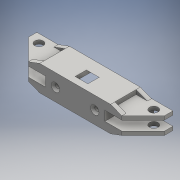
# Autodesk Inventor part: Support_GP2.C
Saved by Autodesk Inventor 2016 (Build 200138000, 138)
## iProperties
Created: 2016-09-29
Part Number: Support_GP2.C
Material: Générique
Document SubType Name: Modeling
Designer: LogOut
Density: 1 g/cm^3
Appearance: Par défaut
Author: LogOut
Autodesk Inventor part; units mm, degrees
ref_plane "YZ Plane" through (0, 0, 0) normal (1, 0, 0) x (0, 1, 0)
ref_plane "XZ Plane" through (0, 0, 0) normal (0, 1, 0) x (-1, 0, 0)
ref_plane "XY Plane" through (0, 0, 0) normal (0, 0, 1) x (1, 0, 0)
sketch "Esquisse1" plane through (0, 0, 0) normal (0, 0, 1) x (1, 0, 0)
  line L0 (-64, 14) -> (64, 14)
  line L1 (64, 14) -> (64, -14)
  line L2 (64, -14) -> (-64, -14)
  line L3 (-64, -14) -> (-64, 14)
  point P0 (0, 0)
  dimension "d0" = 128
  dimension "d1" = 28
  dimension "d2" = 14
  dimension "d3" = 64
  constraints: 8 end point, 2 parallel, 1 horizontal, 1 perpendicular
  measures "d0" distance of L0.start L0.end
  measures "d1" distance of L2.end L0.start
  measures "d2" distance from line of point (0, 0) L0
  measures "d3" distance from line of point (0, 0) L1
extrude "Extrusion1" add sketch "Esquisse1" along normal blind 28
sketch "Esquisse2" plane through (-64, 14, 0) normal (0, 1, 0) x (1, 0, 0)
  line L0 (40, -22) -> (88, -22)
  line L1 (88, -22) -> (88, -6)
  line L2 (88, -6) -> (40, -6)
  line L3 (40, -6) -> (40, -22)
  line L4 (0, 0) -> (128, 0) projected
  line L5 (0, 0) -> (0, -28) projected
  line L6 (128, -28) -> (0, -28) projected
  line L7 (128, 0) -> (128, -28) projected
  point P0 (64, 0)
  dimension "d6" = 40
  dimension "d7" = 48
  dimension "d8" = 40
  dimension "d9" = 6
  dimension "d10" = 6
  dimension "d11" = 16
  constraints: 8 end point, 2 parallel, 1 horizontal, 1 perpendicular
  measures "d6" distance between parallel lines of L5 L3
  measures "d7" distance between parallel lines of L1 L3
  measures "d8" distance between parallel lines of L7 L1
  measures "d9" distance between parallel lines of L4 L2
  measures "d10" distance between parallel lines of L6 L0
  measures "d11" distance of L2.end L0.start
extrude "Extrusion2" cut sketch "Esquisse2" against normal blind 24 contours L3 L2 L1 L0
ref_plane "Plan de construction1" through (-24, 14, 14) normal (0, 0, 1) x (1, 0, 0)
sketch "Esquisse3" plane through (-24, 14, 14) normal (0, 0, 1) x (1, 0, 0)
  line L0 (112.7171, 2) -> (72, 2)
  line L1 (72, 2) -> (52, -18)
  line L2 (-4, -18) -> (-24, 2)
  line L3 (-24, 2) -> (-79.3521, 2)
  line L4 (88, -28) -> (-40, -28) projected
  line L5 (112.7171, 2) -> (112.7171, -53.3012)
  line L6 (112.7171, -53.3012) -> (-79.3521, -53.3012)
  line L7 (-79.3521, -53.3012) -> (-79.3521, 2)
  line L8 (-4, -18) -> (-4, -28)
  line L9 (-40, -28) -> (88, -28) projected
  line L10 (-4, -28) -> (52, -28)
  line L11 (52, -28) -> (52, -18)
  point P0 (24, -14)
  point P1 (54.2399, -28)
  point P2 (-6.2399, -28)
  dimension "d22" = 30
  dimension "d23" = 20
  dimension "d24" = 20
  dimension "d25" = 56
  dimension "d26" = 28
  dimension "d27" = 28
  dimension "d28" = 20
  dimension "d29" = 20
  constraints: 20 end point, 5 perpendicular, 4 point on line, 1 collinear, 1 horizontal, 1 vertical
  measures "d22" distance between parallel lines of L3 L4
  measures "d23" horizontal distance of L2.start L2.end
  measures "d24" horizontal distance of L2.start L2.end
  measures "d25" distance between parallel lines of L11 L8
  measures "d26" distance from line of point (24, -14) L11
  measures "d27" distance from line of point (24, -14) L8
  measures "d28" horizontal distance of L0.end L1.end
  measures "d29" horizontal distance of L0.end L1.end
extrude "Extrusion3" cut sketch "Esquisse3" along normal mid plane 8
sketch "Esquisse4" plane through (0, 0, 28) normal (0, 0, 1) x (1, 0, 0)
  line L0 (88.7171, 16) -> (48, 16)
  line L1 (48, 16) -> (28, -4)
  line L2 (-28, -4) -> (-48, 16)
  line L3 (-48, 16) -> (-103.3521, 16)
  line L4 (88.7171, 16) -> (88.7171, -39.3012)
  line L5 (88.7171, -39.3012) -> (-103.3521, -39.3012)
  line L6 (-103.3521, -39.3012) -> (-103.3521, 16)
  line L7 (-28, -4) -> (-28, -14)
  line L8 (-28, -14) -> (28, -14)
  line L9 (28, -14) -> (28, -4)
  line L10 (-44, -14) -> (-64, 6)
  line L11 (-64, 6) -> (-64, -32.5221)
  line L12 (-64, -32.5221) -> (-44, -32.5221)
  line L13 (-44, -32.5221) -> (-44, -14)
  line L14 (0, 8.6214) -> (0, -9.3191)
  line L15 (-64, -14) -> (64, -14) projected
  line L16 (-64, 14) -> (-64, -14) projected
  line L17 (44, -14) -> (64, 6)
  line L18 (64, 6) -> (64, -32.5221)
  line L19 (64, -32.5221) -> (44, -32.5221)
  line L20 (44, -32.5221) -> (44, -14)
  line L21 (64, -14) -> (-64, -14)
  line L22 (64, 14) -> (64, -14)
  point P0 (0, 0)
  point P1 (0, 0)
  point P2 (30.2399, -14)
  point P3 (-30.2399, -14)
  dimension "d31" = 20
  dimension "d32" = 20
  dimension "d33" = 56
  dimension "d34" = 28
  dimension "d35" = 28
  dimension "d36" = 20
  dimension "d37" = 20
  dimension "d38" = 44
  dimension "d39" = 20
  constraints: 42 end point, 7 symmetric about line, 6 perpendicular, 6 point on line, 4 vertical, 2 collinear, 1 coincident, 1 horizontal
  measures "d31" horizontal distance of L7.start L2.end
  measures "d32" horizontal distance of L7.start L2.end
  measures "d33" distance between parallel lines of L9 L7
  measures "d34" distance from line of point (0, 0) L9
  measures "d35" distance from line of point (0, 0) L7
  measures "d36" horizontal distance of L1.start L9.end
  measures "d37" horizontal distance of L1.start L9.end
  measures "d38" distance between parallel lines of L14 L13
  measures "d39" distance from line of L8 L10.end
extrude "Extrusion4" cut sketch "Esquisse4" against normal through all contours L15 L11 L10 | L13 L12 L11 L15 | L17 L18 L15 | L15 L18 L19 L20
sketch "Esquisse5" plane through (-64, 14, 0) normal (0, 1, 0) x (1, 0, 0)
  line L0 (108, -22) -> (140.1928, -22)
  line L1 (140.1928, -22) -> (140.1928, -6)
  line L2 (140.1928, -6) -> (108, -6)
  line L3 (108, -6) -> (92, 0)
  line L4 (92, 0) -> (36, 0)
  line L5 (20, -6) -> (-10.9625, -6)
  line L6 (-10.9625, -6) -> (-10.9625, -22)
  line L7 (-10.9625, -22) -> (20, -22)
  line L8 (20, -22) -> (36, -28)
  line L9 (36, -28) -> (92, -28)
  line L10 (92, -28) -> (108, -22)
  line L11 (163.0378, -60.3527) -> (-29.6952, -60.3527)
  line L12 (-29.6952, -60.3527) -> (-29.6952, 29.8921)
  line L13 (-29.6952, 29.8921) -> (163.0378, 29.8921)
  line L14 (163.0378, 29.8921) -> (163.0378, -60.3527)
  line L15 (128, -18) -> (110, -18) projected
  line L16 (108, -10) -> (128, -10) projected
  line L17 (128, -28) -> (0, -28) projected
  line L18 (0, 0) -> (128, 0) projected
  line L19 (128, -18) -> (128, -28) projected
  line L20 (0, 0) -> (0, -10) projected
  line L21 (36, 0) -> (20, -6)
  point P0 (64, 0)
  dimension "d42" = 4
  dimension "d43" = 4
  dimension "d44" = 56
  dimension "d45" = 28
  dimension "d46" = 28
  dimension "d47" = 20
  dimension "d48" = 20
  constraints: 32 end point, 6 parallel, 4 perpendicular, 4 point on line, 2 collinear, 2 horizontal
  measures "d42" distance between parallel lines of L15 L0
  measures "d43" distance between parallel lines of L16 L2
  measures "d44" distance of L8.end L9.end
  measures "d45" horizontal distance of point (64, 0) L9.end
  measures "d46" distance of point (64, 0) L3.end
  measures "d47" distance from line of L19 L0.start
  measures "d48" distance from line of L20 L5.start
extrude "Extrusion5" cut sketch "Esquisse5" against normal through all contours L0 L19 L17 L10 | L21 L5 L20 L18 | L11 L12 L13 L14
sketch "Esquisse6" plane through (44, 14, 22) normal (0, 0, 1) x (1, 0, 0)
  line L0 (10, -8) -> (-98, -8)
  line L1 (20, 0) -> (20, -8) projected
  line L2 (-108, -8) -> (-108, 0) projected
  line L3 (-108, 0) -> (-88, 0) projected
  point P0 (-44, -14)
  dimension "d51" = 10
  dimension "d52" = 10
  dimension "d53" = 8
  constraints: 2 end point, 1 horizontal
  measures "d51" distance from line of L1 L0.start
  measures "d52" distance from line of L2 L0.end
  measures "d53" distance between parallel lines of L3 L0
hole "Perçage1" at (54, 6, 22) at (-54, 6, 22) direction (0, 0, -1) diameter 8 end through all
sketch "Esquisse7" plane through (-64, -10, 0) normal (0, 1, 0) x (1, 0, 0)
  line L0 (82.5, -14) -> (45.5, -14)
  line L1 (88, -6) -> (88, -22) projected
  line L2 (40, -6) -> (88, -6) projected
  point P0 (64, 0)
  dimension "d61" = 37
  dimension "d62" = 5.5
  dimension "d63" = 8
  constraints: 2 end point, 1 horizontal
  measures "d61" distance of L0.start L0.end
  measures "d62" distance from line of L1 L0.start
  measures "d63" distance between parallel lines of L0 L2
hole "Perçage2" at (18.5, -10, 14) at (-18.5, -10, 14) direction (0, -1, 0) diameter 4 end through all
chamfer "Chanfrein1" distance 2 angle 45 2 edges at (-18.5, -14, 12) (18.5, -14, 12)
sketch "Esquisse8" plane through (0, 0, 28) normal (0, 0, 1) x (1, 0, 0)
  line L0 (6, -8) -> (-6, -8)
  line L1 (-6, -8) -> (-6, 0)
  line L2 (-6, 0) -> (6, 0)
  line L3 (6, 0) -> (6, -8)
  line L4 (-28, -14) -> (28, -14) projected
  point P0 (0, 0)
  dimension "d74" = 12
  dimension "d75" = 8
  dimension "d76" = 6
  dimension "d77" = 6
  constraints: 8 end point, 2 parallel, 1 horizontal, 1 perpendicular
  measures "d74" distance of L0.start L0.end
  measures "d75" distance between parallel lines of L0 L2
  measures "d76" distance between parallel lines of L4 L0
  measures "d77" distance from line of point (0, 0) L3
extrude "Extrusion6" cut sketch "Esquisse8" against normal blind 6
chamfer "Chanfrein2" distance 8 distance2 6 1 edges at (0, 0, 22) measured on face at (0, 0.5, 22)
sketch "Esquisse9" plane through (0, 0, 28) normal (0, 0, 1) x (1, 0, 0)
  line L0 (44, -14) -> (28, -14) projected
  line L1 (44, 14) -> (44, -14) projected
  line L2 (28, 14) -> (44, 14) projected
  line L3 (28, -14) -> (28, 14) projected
  line L4 (-28, -14) -> (-44, -14) projected
  line L5 (-28, 14) -> (-28, -14) projected
  line L6 (-44, 14) -> (-28, 14) projected
  line L7 (-44, 14) -> (-44, -14) projected
  line L8 (44, -10) -> (28, -10)
  line L9 (28, -4) -> (28, -14) projected
  line L10 (28, -14) -> (28, 14) projected
  line L11 (28, 10) -> (44, 10)
  line L12 (44, 14) -> (44, -14) projected
  line L13 (0, -3.5087) -> (0, 10)
  line L14 (-44, -14) -> (-28, -14)
  line L15 (-44, 14) -> (-44, -14)
  line L16 (-28, 14) -> (-44, 14)
  line L17 (-28, -14) -> (-28, 14)
  line L18 (-44, -10) -> (-28, -10)
  line L19 (-28, -4) -> (-28, -14)
  line L20 (-28, -14) -> (-28, 14)
  line L21 (-28, 10) -> (-44, 10)
  line L22 (-44, 14) -> (-44, -14)
  point P0 (0, 0)
  dimension "d83" = 4
  dimension "d84" = 4
  constraints: 24 end point, 8 point on line, 5 symmetric about line, 1 parallel, 1 perpendicular, 1 vertical
  measures "d83" distance between parallel lines of L2 L11
  measures "d84" distance between parallel lines of L0 L8
extrude "Extrusion7" cut sketch "Esquisse9" against normal blind 6 contours L8 L3 L11 L1 | L18 L7 L21 L5
mirror "Symétrie1" about plane through (-24, 14, 14) normal (0, 0, 1) of "Extrusion7"
move faces "Déplacer1" translate (0, 0, 0.5) faces at (-40.9027, -4.7574, 18) (40.9027, -4.7574, 18)
move faces "Déplacer2" translate (0, 0, -0.5) faces at (-40.9027, -4.7574, 10) (40.9027, -4.7574, 10)
move faces "Déplacer3" translate (0, 0, -2) faces at (2, 9.3333, 28)
move faces "Déplacer4" translate (0, 0, 2) faces at (-9.0363, 5.0363, 0)
chamfer "Chanfrein4" distance 10 distance2 24 1 edges at (24, 14, 14) measured on face at (24.5, 14, 14)
chamfer "Chanfrein5" distance 10 distance2 24 1 edges at (-24, 14, 14) measured on face at (-24.5, 14, 14)
move faces "Déplacer5" translate (5.3333, 0, 0) faces at (28, -0.1333, 3.3333) (28, 6.5333, 23.3333)
move faces "Déplacer6" translate (-5.3333, 0, 0) faces at (-28, -0.1333, 3.3333) (-28, 6.5333, 23.3333)
chamfer "Chanfrein6" distance 2 angle 45 2 edges at (0, 14, 6) (0, 14, 22)
